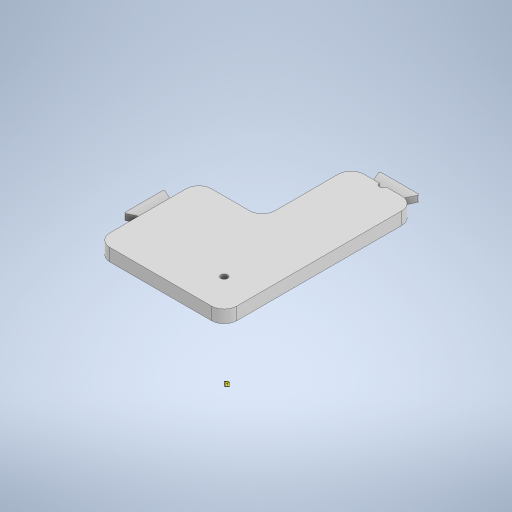
# Autodesk Inventor part: Area nv
Saved by Autodesk Inventor 2024 (Build 280153000, 153)
## iProperties
Created: 2024-03-01
Part Number: Area nv
Material: Generic
Document SubType Name: Modeling
Designer: laura
Density: 1 g/cm^3
Appearance: Default
Author: laura
Autodesk Inventor part; units mm, degrees
ref_plane "YZ Plane" through (0, 0, 0) normal (1, 0, 0) x (0, 1, 0)
ref_plane "XZ Plane" through (0, 0, 0) normal (0, 1, 0) x (-1, 0, 0)
ref_plane "XY Plane" through (0, 0, 0) normal (0, 0, 1) x (1, 0, 0)
sketch "Sketch1" plane through (0, 0, 0) normal (0, 1, 0) x (-1, 0, 0)
  line L0 (0, 0) -> (150, 0)
  line L1 (150, 0) -> (150, -200)
  line L2 (150, -200) -> (0, -200)
  line L3 (0, -200) -> (0, 0)
  line L4 (150, -200) -> (150, -143.8709)
  dimension "d0" = 150
  dimension "d1" = 200
  constraints: 10 end point, 2 parallel, 1 horizontal, 1 perpendicular, 1 point on line
  measures "d0" distance of L1.end L2.end
  measures "d1" distance of L0.end L1.end
extrude "Extrusion1" add sketch "Sketch1" along normal blind 10
sketch "Sketch3" plane through (0, 0, 0) normal (0, -1, 0) x (1, 0, 0)
  line L0 (-85, -199.8) -> (-85, -213.2303) construction
  line L1 (0, -200) -> (-150, -200) projected
  line L2 (-75, -213.1946) -> (-89.7696, -213.1946)
  arc A0 (-90.4946, -212.0565) -> (-89.7696, -213.1946) centre (-89.7696, -212.3946) ccw
  line L3 (-90.4946, -212.0565) -> (-84.8726, -200)
  line L4 (-84.8726, -200) -> (-65.1274, -200)
  line L5 (-65.1274, -200) -> (-59.5054, -212.0565)
  arc A1 (-60.2304, -213.1946) -> (-59.5054, -212.0565) centre (-60.2304, -212.3946) ccw
  line L6 (-60.2304, -213.1946) -> (-75, -213.1946)
  line L7 (-149.8, -90) -> (-163.2303, -90) construction
  line L8 (-163.1946, -100) -> (-163.1946, -85.2304)
  arc A2 (-162.0565, -84.5054) -> (-163.1946, -85.2304) centre (-162.3946, -85.2304) ccw
  line L9 (-162.0565, -84.5054) -> (-150, -90.1274)
  line L10 (-150, -90.1274) -> (-150, -109.8726)
  line L11 (-150, -109.8726) -> (-162.0565, -115.4946)
  arc A3 (-163.1946, -114.7696) -> (-162.0565, -115.4946) centre (-162.3946, -114.7696) ccw
  line L12 (-163.1946, -114.7696) -> (-163.1946, -100)
  line L13 (-150, -200) -> (-150, 0) projected
  point P0 (0, 0)
  point P1 (-75, -200)
  point P2 (-75, -200)
  point P3 (-150, -100)
  point P4 (-150, -100)
  point P5 (-150, -100)
  constraints: 24 end point, 8 point on circle, 4 centre point, 3 midpoint
extrude "Extrusion3" add sketch "Sketch3" against normal blind 4.8
sketch "Sketch5" plane through (0, 10, 0) normal (0, 1, 0) x (1, 0, 0)
  line L0 (-150, 200) -> (-150, 0) projected
  line L1 (-150, 0) -> (-75, 0)
  line L2 (-150, 0) -> (0, 0) projected
  line L3 (-75, 0) -> (-75, 75)
  circle A0 centre (-75, 75) radius 2.5
  circle A1 centre (-75, 75) radius 2.6
  line L4 (-150, 200) -> (-150, 0) projected
  line L5 (-150, 200) -> (-75, 200)
  line L6 (0, 200) -> (-150, 200) projected
  circle A2 centre (-75, 200) radius 2.5
  circle A3 centre (-75, 200) radius 2.6
  point P0 (-150, 89.7793)
  point P1 (-150, 110.2207)
  dimension "d17" = 75
  dimension "d18" = 5
  dimension "d19" = 0.1
  dimension "d20" = 5
  dimension "d21" = 0.1
  constraints: 6 end point, 4 centre point, 2 coincident, 2 midpoint, 1 vertical
  measures "d17" distance of L1.end L3.end
  measures "d18" diameter of A0
  measures "d19" radial gap between concentric circles of A0 A1
  measures "d20" diameter of A2
  measures "d21" radial gap between concentric circles of A2 A3
extrude "Extrusion4" cut sketch "Sketch5" against normal blind 5.2 contours A0 | A1 | A3 L6 A2 L5 | L5 A2 L6 A3 | A2 L6 L5 | L5 L6 A2
sketch "Sketch7" plane through (0, 10, 0) normal (0, 1, 0) x (1, 0, 0)
  line L0 (0, 0) -> (0, 200) projected
  line L1 (-150, 0) -> (0, 0) projected
  line L2 (0, 200) -> (-50, 200)
  line L3 (-50, 200) -> (-50, 0)
  line L4 (-50, 0) -> (0, 0)
  line L5 (0, 0) -> (0, 200)
  line L6 (-150, 0) -> (0, 0)
  line L7 (0, 0) -> (0, 50)
  line L8 (0, 50) -> (-150, 50)
  line L9 (-150, 50) -> (-150, 0)
  line L10 (-150, 200) -> (-100, 200)
  line L11 (-100, 200) -> (-100, 130)
  line L12 (-100, 130) -> (-150, 130)
  line L13 (-150, 130) -> (-150, 200)
  point P0 (-50, 50)
  dimension "d24" = 50
  dimension "d25" = 50
  dimension "d26" = 50
  dimension "d27" = 70
  constraints: 24 end point, 6 parallel, 4 point on line, 3 horizontal, 3 perpendicular
  measures "d24" distance of L4.end L3.end
  measures "d25" distance of L7.end L6.end
  measures "d26" distance of L11.end L12.end
  measures "d27" distance of L10.end L11.end
extrude "Extrusion5" cut sketch "Sketch7" against normal blind 10
fillet "Fillet1" radius 10 6 edges at (-50, 5, -200) (-100, 5, -200) (-150, 5, -130) (-100, 5, -130) (-50, 5, -50) (-150, 5, -50)
body "Solid1"
